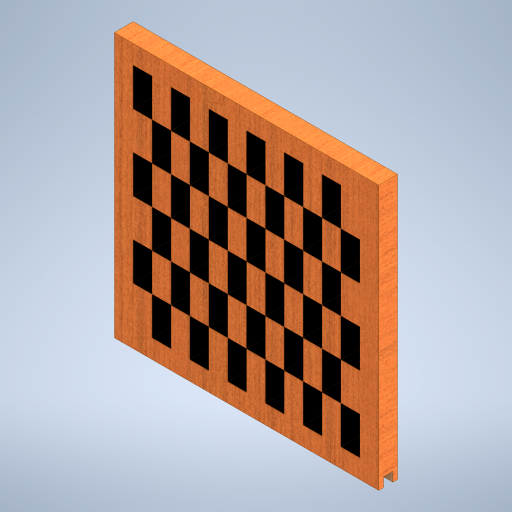
# Autodesk Inventor part: JukeBox Outside panel sharp edges magnet slit
Saved by Autodesk Inventor 2024 (Build 280153000, 153)
## iProperties
Created: 2023-04-22
Part Number: JukeBox Outside panel sharp edges magnet slit
Material: Oak, Red
Document SubType Name: Modeling
Designer: newic
Density: 0.673 g/cm^3
Appearance: Cherry - Natural Low Gloss
Author: newic
Autodesk Inventor part; units mm, degrees
ref_plane "YZ Plane" through (0, 0, 0) normal (1, 0, 0) x (0, 1, 0)
ref_plane "XZ Plane" through (0, 0, 0) normal (0, 1, 0) x (-1, 0, 0)
ref_plane "XY Plane" through (0, 0, 0) normal (0, 0, 1) x (1, 0, 0)
sketch "Sketch1" plane through (0, 0, 0) normal (0, 0, 1) x (1, 0, 0)
  line L0 (0, 0) -> (812.8, 0) construction
  line L1 (812.8, 0) -> (812.8, -406.4) construction
  line L2 (812.8, -406.4) -> (0, -406.4) construction
  line L3 (0, -406.4) -> (0, 0) construction
  line L4 (0, 0) -> (406.4, 0)
  line L5 (406.4, 0) -> (406.4, -25.4)
  line L6 (406.4, -25.4) -> (0, -25.4)
  line L7 (0, -25.4) -> (0, 0)
  line L8 (406.4, -25.4) -> (381, -25.4)
  line L9 (381, -25.4) -> (381, -406.4)
  line L10 (381, -406.4) -> (406.4, -406.4)
  line L11 (406.4, -406.4) -> (406.4, -25.4)
  line L12 (381, -406.4) -> (0, -406.4)
  line L13 (0, -406.4) -> (0, -381)
  line L14 (0, -381) -> (381, -381)
  line L15 (381, -381) -> (381, -406.4)
  line L16 (0, -381) -> (25.4, -381)
  line L17 (25.4, -381) -> (25.4, -25.4)
  line L18 (25.4, -25.4) -> (0, -25.4)
  line L19 (0, -25.4) -> (0, -381)
  dimension "d1" = 812.8
  dimension "d5" = 406.4
  dimension "d6" = 25.4
  dimension "d7" = 25.4
  dimension "d8" = 381
  dimension "d9" = 381
  dimension "d10" = 25.4
  dimension "d11" = 25.4
  constraints: 32 end point, 8 parallel, 4 horizontal, 4 perpendicular, 1 point on line, 2 other
  measures "d1" distance of L1.end L2.end
  measures "d5" distance of L5.end L6.end
  measures "d6" distance of L4.end L5.end
  measures "d7" distance of L10.end L9.end
  measures "d8" distance of L9.end L8.end
  measures "d9" distance of L13.end L14.end
  measures "d10" distance of L12.end L13.end
  measures "d11" distance of L18.end L17.end
extrude "Extrusion1" add sketch "Sketch1" against normal blind 25.4 contours L6 L9 L14 L17
sketch "Sketch2" plane through (0, 0, 0) normal (0, 0, 1) x (1, 0, 0)
  line L0 (0, 0) -> (812.8, 0) construction
  line L1 (812.8, 0) -> (812.8, -406.4) construction
  line L2 (812.8, -406.4) -> (0, -406.4) construction
  line L3 (0, -406.4) -> (0, 0) construction
  line L4 (25.4, -25.4) -> (381, -25.4) projected
  line L5 (25.4, -25.4) -> (50.8, -25.4)
  line L6 (50.8, -25.4) -> (50.8, -50.8)
  line L7 (50.8, -50.8) -> (25.4, -50.8)
  line L8 (25.4, -50.8) -> (25.4, -25.4)
  line L9 (50.8, -50.8) -> (76.2, -50.8)
  line L10 (76.2, -50.8) -> (76.2, -101.6)
  line L11 (76.2, -101.6) -> (50.8, -101.6)
  line L12 (50.8, -101.6) -> (50.8, -50.8)
  line L13 (76.2, -101.6) -> (101.6, -101.6)
  line L14 (101.6, -101.6) -> (101.6, -152.4)
  line L15 (101.6, -152.4) -> (76.2, -152.4)
  line L16 (76.2, -152.4) -> (76.2, -101.6)
  line L17 (101.6, -152.4) -> (127, -152.4)
  line L18 (127, -152.4) -> (127, -203.2)
  line L19 (127, -203.2) -> (101.6, -203.2)
  line L20 (101.6, -203.2) -> (101.6, -152.4)
  line L21 (127, -203.2) -> (152.4, -203.2)
  line L22 (152.4, -203.2) -> (152.4, -254)
  line L23 (152.4, -254) -> (127, -254)
  line L24 (127, -254) -> (127, -203.2)
  line L25 (152.4, -254) -> (177.8, -254)
  line L26 (177.8, -254) -> (177.8, -304.8)
  line L27 (177.8, -304.8) -> (152.4, -304.8)
  line L28 (152.4, -304.8) -> (152.4, -254)
  line L29 (177.8, -304.8) -> (203.2, -304.8)
  line L30 (203.2, -304.8) -> (203.2, -355.6)
  line L31 (203.2, -355.6) -> (177.8, -355.6)
  line L32 (177.8, -355.6) -> (177.8, -304.8)
  line L33 (50.8, -152.4) -> (76.2, -152.4)
  line L34 (76.2, -152.4) -> (76.2, -203.2)
  line L35 (76.2, -203.2) -> (50.8, -203.2)
  line L36 (50.8, -203.2) -> (50.8, -152.4)
  line L37 (76.2, -203.2) -> (101.6, -203.2)
  line L38 (101.6, -203.2) -> (101.6, -254)
  line L39 (101.6, -254) -> (76.2, -254)
  line L40 (76.2, -254) -> (76.2, -203.2)
  line L41 (101.6, -254) -> (127, -254)
  line L42 (127, -254) -> (127, -304.8)
  line L43 (127, -304.8) -> (101.6, -304.8)
  line L44 (101.6, -304.8) -> (101.6, -254)
  line L45 (127, -304.8) -> (152.4, -304.8)
  line L46 (152.4, -304.8) -> (152.4, -355.6)
  line L47 (152.4, -355.6) -> (127, -355.6)
  line L48 (127, -355.6) -> (127, -304.8)
  line L49 (50.8, -254) -> (76.2, -254)
  line L50 (76.2, -254) -> (76.2, -304.8)
  line L51 (76.2, -304.8) -> (50.8, -304.8)
  line L52 (50.8, -304.8) -> (50.8, -254)
  line L53 (76.2, -304.8) -> (101.6, -304.8)
  line L54 (101.6, -304.8) -> (101.6, -355.6)
  line L55 (101.6, -355.6) -> (76.2, -355.6)
  line L56 (76.2, -355.6) -> (76.2, -304.8)
  line L57 (203.2, -254) -> (228.6, -254)
  line L58 (228.6, -254) -> (228.6, -304.8)
  line L59 (228.6, -304.8) -> (203.2, -304.8)
  line L60 (203.2, -304.8) -> (203.2, -254)
  line L61 (228.6, -304.8) -> (254, -304.8)
  line L62 (254, -304.8) -> (254, -355.6)
  line L63 (254, -355.6) -> (228.6, -355.6)
  line L64 (228.6, -355.6) -> (228.6, -304.8)
  line L65 (152.4, -152.4) -> (177.8, -152.4)
  line L66 (177.8, -152.4) -> (177.8, -203.2)
  line L67 (177.8, -203.2) -> (152.4, -203.2)
  line L68 (152.4, -203.2) -> (152.4, -152.4)
  line L69 (177.8, -203.2) -> (203.2, -203.2)
  line L70 (203.2, -203.2) -> (203.2, -254)
  line L71 (203.2, -254) -> (177.8, -254)
  line L72 (177.8, -254) -> (177.8, -203.2)
  line L73 (101.6, -50.8) -> (127, -50.8)
  line L74 (127, -50.8) -> (127, -101.6)
  line L75 (127, -101.6) -> (101.6, -101.6)
  line L76 (101.6, -101.6) -> (101.6, -50.8)
  line L77 (127, -101.6) -> (152.4, -101.6)
  line L78 (152.4, -101.6) -> (152.4, -152.4)
  line L79 (152.4, -152.4) -> (127, -152.4)
  line L80 (127, -152.4) -> (127, -101.6)
  line L81 (254, -254) -> (279.4, -254)
  line L82 (279.4, -254) -> (279.4, -304.8)
  line L83 (279.4, -304.8) -> (254, -304.8)
  line L84 (254, -304.8) -> (254, -254)
  line L85 (279.4, -304.8) -> (304.8, -304.8)
  line L86 (304.8, -304.8) -> (304.8, -355.6)
  line L87 (304.8, -355.6) -> (279.4, -355.6)
  line L88 (279.4, -355.6) -> (279.4, -304.8)
  line L89 (203.2, -152.4) -> (228.6, -152.4)
  line L90 (228.6, -152.4) -> (228.6, -203.2)
  line L91 (228.6, -203.2) -> (203.2, -203.2)
  line L92 (203.2, -203.2) -> (203.2, -152.4)
  line L93 (228.6, -203.2) -> (254, -203.2)
  line L94 (254, -203.2) -> (254, -254)
  line L95 (254, -254) -> (228.6, -254)
  line L96 (228.6, -254) -> (228.6, -203.2)
  line L97 (152.4, -50.8) -> (177.8, -50.8)
  line L98 (177.8, -50.8) -> (177.8, -101.6)
  line L99 (177.8, -101.6) -> (152.4, -101.6)
  line L100 (152.4, -101.6) -> (152.4, -50.8)
  line L101 (177.8, -101.6) -> (203.2, -101.6)
  line L102 (203.2, -101.6) -> (203.2, -152.4)
  line L103 (203.2, -152.4) -> (177.8, -152.4)
  line L104 (177.8, -152.4) -> (177.8, -101.6)
  line L105 (304.8, -254) -> (330.2, -254)
  line L106 (330.2, -254) -> (330.2, -304.8)
  line L107 (330.2, -304.8) -> (304.8, -304.8)
  line L108 (304.8, -304.8) -> (304.8, -254)
  line L109 (330.2, -304.8) -> (355.6, -304.8)
  line L110 (355.6, -304.8) -> (355.6, -355.6)
  line L111 (355.6, -355.6) -> (330.2, -355.6)
  line L112 (330.2, -355.6) -> (330.2, -304.8)
  line L113 (254, -152.4) -> (279.4, -152.4)
  line L114 (279.4, -152.4) -> (279.4, -203.2)
  line L115 (279.4, -203.2) -> (254, -203.2)
  line L116 (254, -203.2) -> (254, -152.4)
  line L117 (279.4, -203.2) -> (304.8, -203.2)
  line L118 (304.8, -203.2) -> (304.8, -254)
  line L119 (304.8, -254) -> (279.4, -254)
  line L120 (279.4, -254) -> (279.4, -203.2)
  line L121 (203.2, -50.8) -> (228.6, -50.8)
  line L122 (228.6, -50.8) -> (228.6, -101.6)
  line L123 (228.6, -101.6) -> (203.2, -101.6)
  line L124 (203.2, -101.6) -> (203.2, -50.8)
  line L125 (228.6, -101.6) -> (254, -101.6)
  line L126 (254, -101.6) -> (254, -152.4)
  line L127 (254, -152.4) -> (228.6, -152.4)
  line L128 (228.6, -152.4) -> (228.6, -101.6)
  line L129 (304.8, -152.4) -> (330.2, -152.4)
  line L130 (330.2, -152.4) -> (330.2, -203.2)
  line L131 (330.2, -203.2) -> (304.8, -203.2)
  line L132 (304.8, -203.2) -> (304.8, -152.4)
  line L133 (330.2, -203.2) -> (355.6, -203.2)
  line L134 (355.6, -203.2) -> (355.6, -254)
  line L135 (355.6, -254) -> (330.2, -254)
  line L136 (330.2, -254) -> (330.2, -203.2)
  line L137 (254, -50.8) -> (279.4, -50.8)
  line L138 (279.4, -50.8) -> (279.4, -101.6)
  line L139 (279.4, -101.6) -> (254, -101.6)
  line L140 (254, -101.6) -> (254, -50.8)
  line L141 (279.4, -101.6) -> (304.8, -101.6)
  line L142 (304.8, -101.6) -> (304.8, -152.4)
  line L143 (304.8, -152.4) -> (279.4, -152.4)
  line L144 (279.4, -152.4) -> (279.4, -101.6)
  line L145 (304.8, -50.8) -> (330.2, -50.8)
  line L146 (330.2, -50.8) -> (330.2, -101.6)
  line L147 (330.2, -101.6) -> (304.8, -101.6)
  line L148 (304.8, -101.6) -> (304.8, -50.8)
  line L149 (330.2, -101.6) -> (355.6, -101.6)
  line L150 (355.6, -101.6) -> (355.6, -152.4)
  line L151 (355.6, -152.4) -> (330.2, -152.4)
  line L152 (330.2, -152.4) -> (330.2, -101.6)
  dimension "d15" = 812.8
  dimension "d19" = 25.4
  dimension "d20" = 25.4
  dimension "d21" = 25.4
  dimension "d22" = 50.8
  dimension "d23" = 25.4
  dimension "d24" = 50.8
  dimension "d25" = 25.4
  dimension "d26" = 50.8
  dimension "d27" = 25.4
  dimension "d28" = 50.8
  dimension "d30" = 25.4
  dimension "d31" = 50.8
  dimension "d32" = 25.4
  dimension "d33" = 50.8
  dimension "d35" = 25.4
  dimension "d36" = 50.8
  dimension "d37" = 25.4
  dimension "d38" = 50.8
  dimension "d40" = 25.4
  dimension "d41" = 50.8
  dimension "d42" = 25.4
  dimension "d43" = 50.8
  dimension "d45" = 25.4
  dimension "d46" = 50.8
  dimension "d47" = 25.4
  dimension "d48" = 50.8
  dimension "d50" = 25.4
  dimension "d51" = 50.8
  dimension "d52" = 25.4
  dimension "d53" = 50.8
  dimension "d55" = 25.4
  dimension "d56" = 50.8
  dimension "d57" = 25.4
  dimension "d58" = 50.8
  dimension "d60" = 25.4
  dimension "d61" = 50.8
  dimension "d62" = 25.4
  dimension "d63" = 50.8
  dimension "d65" = 25.4
  dimension "d66" = 50.8
  dimension "d67" = 25.4
  dimension "d68" = 50.8
  dimension "d70" = 25.4
  dimension "d71" = 50.8
  dimension "d72" = 25.4
  dimension "d73" = 50.8
  dimension "d75" = 25.4
  dimension "d76" = 50.8
  dimension "d77" = 25.4
  dimension "d78" = 50.8
  dimension "d80" = 25.4
  dimension "d81" = 50.8
  dimension "d82" = 25.4
  dimension "d83" = 50.8
  dimension "d85" = 25.4
  dimension "d86" = 50.8
  dimension "d87" = 25.4
  dimension "d88" = 50.8
  dimension "d90" = 25.4
  dimension "d91" = 50.8
  dimension "d92" = 25.4
  dimension "d93" = 50.8
  dimension "d95" = 25.4
  constraints: 296 end point, 74 parallel, 37 horizontal, 37 perpendicular, 2 other
  measures "d15" distance of L1.end L2.end
  measures "d19" distance of L6.end L7.end
  measures "d20" distance of L5.end L6.end
  measures "d21" distance of L10.end L11.end
  measures "d22" distance of L9.end L10.end
  measures "d23" distance of L14.end L15.end
  measures "d24" distance of L13.end L14.end
  measures "d25" distance of L19.start L19.end
  measures "d26" distance of L18.start L19.start
  measures "d27" distance of L22.end L24.start
  measures "d28" distance of L21.end L22.end
  measures "d30" distance of L27.start L27.end
  measures "d31" distance of L26.start L27.start
  measures "d32" distance of L30.end L32.start
  measures "d33" distance of L29.end L30.end
  measures "d35" distance of L35.start L35.end
  measures "d36" distance of L34.start L35.start
  measures "d37" distance of L38.end L40.start
  measures "d38" distance of L37.end L38.end
  measures "d40" distance of L43.start L43.end
  measures "d41" distance of L42.start L43.start
  measures "d42" distance of L46.end L48.start
  measures "d43" distance of L45.end L46.end
  measures "d45" distance of L51.start L51.end
  measures "d46" distance of L50.start L51.start
  measures "d47" distance of L54.end L56.start
  measures "d48" distance of L53.end L54.end
  measures "d50" distance of L59.start L59.end
  measures "d51" distance of L58.start L59.start
  measures "d52" distance of L62.end L64.start
  measures "d53" distance of L61.end L62.end
  measures "d55" distance of L67.start L67.end
  measures "d56" distance of L66.start L67.start
  measures "d57" distance of L70.end L72.start
  measures "d58" distance of L69.end L70.end
  measures "d60" distance of L75.start L75.end
  measures "d61" distance of L74.start L75.start
  measures "d62" distance of L78.end L80.start
  measures "d63" distance of L77.end L78.end
  measures "d65" distance of L83.start L83.end
  measures "d66" distance of L82.start L83.start
  measures "d67" distance of L86.end L88.start
  measures "d68" distance of L85.end L86.end
  measures "d70" distance of L91.start L91.end
  measures "d71" distance of L90.start L91.start
  measures "d72" distance of L94.end L96.start
  measures "d73" distance of L93.end L94.end
  measures "d75" distance of L99.start L99.end
  measures "d76" distance of L98.start L99.start
  measures "d77" distance of L102.end L104.start
  measures "d78" distance of L101.end L102.end
  measures "d80" distance of L107.start L107.end
  measures "d81" distance of L106.start L107.start
  measures "d82" distance of L110.end L112.start
  measures "d83" distance of L109.end L110.end
  measures "d85" distance of L115.start L115.end
  measures "d86" distance of L114.start L115.start
  measures "d87" distance of L118.end L120.start
  measures "d88" distance of L117.end L118.end
  measures "d90" distance of L123.start L123.end
  measures "d91" distance of L122.start L123.start
  measures "d92" distance of L126.end L128.start
  measures "d93" distance of L125.end L126.end
  measures "d95" distance of L131.start L131.end
extrude "Extrusion2" cut sketch "Sketch2" against normal blind 50.8 contours L109 L110 L111 L112 | L13 L14 L15 L16 | L9 L10 L11 L12 | L76 L73 L74 L75 | L34 L35 L36 L33 | L17 L18 L19 L20 | L77 L78 L79 L80 | L37 L38 L39 L40 | L100 L97 L98 L99 | L50 L51 L52 L49 | L21 L22 L23 L24 | L65 L66 L67 L68 | L41 L42 L43 L44 | L101 L102 L103 L104 | L53 L54 L55 L56 | L124 L121 L122 L123 | L25 L26 L27 L28 | L69 L70 L71 L72 | L45 L46 L47 L48 | L89 L90 L91 L92 | L125 L126 L127 L128 | L140 L137 L138 L139 | L29 L30 L31 L32 | L57 L58 L59 L60 | L93 L94 L95 L96 | L113 L114 L115 L116 | L141 L142 L143 L144 | L148 L145 L146 L147 | L61 L62 L63 L64 | L81 L82 L83 L84 | L117 L118 L119 L120 | L129 L130 L131 L132 | L149 L150 L151 L152 | L85 L86 L87 L88 | L105 L106 L107 L108 | L133 L134 L135 L136
sketch "Sketch3" plane through (25.4, -381, 0) normal (0, -1, 0) x (1, 0, 0)
  line L0 (0, 0) -> (0, -25.4) projected
  line L1 (0, 0) -> (14.1729, 0)
  line L2 (14.1729, 0) -> (14.1729, -12.7)
  line L3 (14.1729, -12.7) -> (0, -12.7)
  line L4 (0, -12.7) -> (0, 0)
  line L5 (0, -12.7) -> (14.1729, -12.7)
  line L6 (14.1729, -12.7) -> (14.1729, -6.35)
  line L7 (14.1729, -6.35) -> (0, -6.35)
  line L8 (0, -6.35) -> (0, -12.7)
  line L9 (355.6, -25.4) -> (0, -25.4) projected
  line L10 (0, -12.7) -> (14.1729, -12.7)
  line L11 (14.1729, -12.7) -> (14.1729, -25.4)
  line L12 (14.1729, -25.4) -> (0, -25.4)
  line L13 (0, -25.4) -> (0, -12.7)
  line L14 (0, -6.35) -> (355.6, -6.35)
  line L15 (355.6, -6.35) -> (355.6, -19.05)
  line L16 (355.6, -19.05) -> (0, -19.05)
  line L17 (0, -19.05) -> (0, -6.35)
  point P0 (-25.4, 0)
  point P1 (0, -19.05)
  constraints: 32 end point, 8 parallel, 4 horizontal, 4 perpendicular, 2 point on line, 1 midpoint
extrude "Extrusion3" cut sketch "Sketch3" against normal blind 12.7 contours L7 L2 L3 L0 | L3 L11 L16 L0 | L14 L15 L16 L11 L2
body "Solid1"
